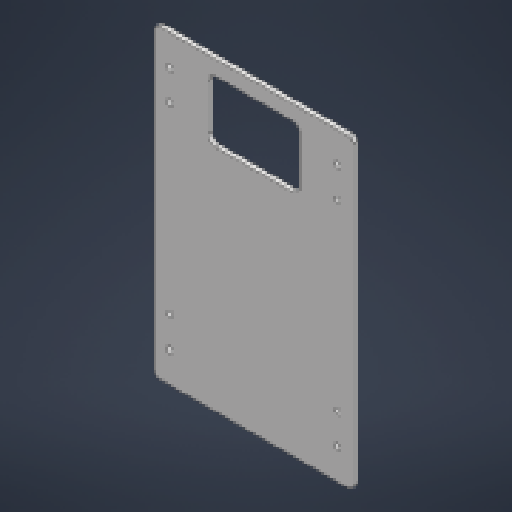
# Autodesk Inventor part: 顶板装配隔离
Saved by Autodesk Inventor 2025 (Build 290162000, 162)
## iProperties
Created: 2026-01-03
Part Number: 顶板装配隔离
Material: 常规
Document SubType Name: Modeling
Designer: XH
Density: 1 g/cm^3
Appearance: 默认
Author: XH
Autodesk Inventor part; units mm, degrees
ref_plane "YZ Plane" through (0, 0, 0) normal (1, 0, 0) x (0, 1, 0)
ref_plane "XZ Plane" through (0, 0, 0) normal (0, 1, 0) x (-1, 0, 0)
ref_plane "XY Plane" through (0, 0, 0) normal (0, 0, 1) x (1, 0, 0)
sketch "草图1" plane through (0, 0, 0) normal (0, 0, 1) x (1, 0, 0)
  line L0 (65, -50) -> (-65, -50)
  line L1 (-65, -50) -> (-65, 50)
  line L2 (-65, 50) -> (65, 50)
  line L3 (65, 50) -> (65, -50)
  line L4 (65, -50) -> (-65, 50) construction
  line L5 (-65, -50) -> (65, 50) construction
  point P0 (0, 0)
  dimension "d0" = 130
  dimension "d1" = 100
  constraints: 12 end point, 2 midpoint, 2 parallel, 1 horizontal, 1 perpendicular
  measures "d0" distance of L1.end L2.end
  measures "d1" distance of L2.end L0.start
extrude "拉伸1" add sketch "草图1" along normal blind 3
fillet "圆角1" radius 3 4 edges at (65, 50, 1.5) (65, -50, 1.5) (-65, -50, 1.5) (-65, 50, 1.5)
sketch "草图2" plane through (0, 0, 0) normal (0, 0, -1) x (-1, 0, 0)
  point P0 (0, 0)
move faces "移动1" translate (0, 50, 0) faces at (20.6667, 50, 1)
move faces "移动2" translate (0, -50, 0) faces at (-20.6667, -50, 1)
sketch "草图3" plane through (0, 0, 0) normal (0, 0, -1) x (-1, 0, 0)
  circle A0 centre (-51, -3) radius 2 projected
  circle A1 centre (51, -3) radius 2 projected
  arc A2 (35, -95) -> (40, -100) centre (40, -95) ccw projected
  line L0 (35, -95) -> (35, -55) projected
  arc A3 (35, -55) -> (30, -50) centre (30, -55) ccw projected
  line L1 (30, -50) -> (-30, -50) projected
  arc A4 (-30, -50) -> (-35, -55) centre (-30, -55) ccw projected
  line L2 (-35, -55) -> (-35, -95) projected
  arc A5 (-40, -100) -> (-35, -95) centre (-40, -95) ccw projected
  line L3 (-65, -100) -> (-40, -100) projected
  line L4 (-65, -20) -> (-65, -100) projected
  line L5 (-65, -20) -> (-120, -20) projected
  line L6 (-120, -20) -> (-120, 20) projected
  line L7 (-120, 20) -> (-65, 20) projected
  line L8 (-65, 100) -> (-65, 20) projected
  line L9 (65, 100) -> (-65, 100) projected
  line L10 (65, 20) -> (65, 100) projected
  line L11 (65, 20) -> (120, 20) projected
  line L12 (120, 20) -> (120, -20) projected
  line L13 (120, -20) -> (65, -20) projected
  line L14 (65, -100) -> (65, -20) projected
  line L15 (40, -100) -> (65, -100) projected
  line L16 (-25, 50) -> (25, 50) projected
  arc A6 (25, 50) -> (30, 55) centre (25, 55) ccw projected
  line L17 (30, 55) -> (30, 85) projected
  arc A7 (30, 85) -> (25, 90) centre (25, 85) ccw projected
  line L18 (25, 90) -> (-25, 90) projected
  arc A8 (-25, 90) -> (-30, 85) centre (-25, 85) ccw projected
  line L19 (-30, 85) -> (-30, 55) projected
  arc A9 (-30, 55) -> (-25, 50) centre (-25, 55) ccw projected
  circle A10 centre (-106, -10) radius 2.5 projected
  circle A11 centre (86, 10) radius 2.5 projected
  circle A12 centre (-86, -10) radius 2.5 projected
  circle A13 centre (-86, 10) radius 2.5 projected
  circle A14 centre (106, -10) radius 2.5 projected
  circle A15 centre (106, 10) radius 2.5 projected
  circle A16 centre (-106, 10) radius 2.5 projected
  circle A17 centre (86, -10) radius 2.5 projected
  line L20 (-8.0092, 23.9084) -> (-13.0092, 23.9084) projected
  line L21 (-13.0092, 23.9084) -> (-13.0092, 18.9084) projected
  line L22 (-13.0092, 18.9084) -> (-8.0092, 18.9084) projected
  line L23 (-8.0092, 18.9084) -> (-8.0092, 23.9084) projected
  line L24 (-23.0092, 23.9084) -> (-28.0092, 23.9084) projected
  line L25 (-28.0092, 23.9084) -> (-28.0092, 18.9084) projected
  line L26 (-28.0092, 18.9084) -> (-23.0092, 18.9084) projected
  line L27 (-23.0092, 18.9084) -> (-23.0092, 23.9084) projected
  line L28 (-8.0092, -26.0916) -> (-13.0092, -26.0916) projected
  line L29 (-13.0092, -26.0916) -> (-13.0092, -31.0916) projected
  line L30 (-13.0092, -31.0916) -> (-8.0092, -31.0916) projected
  line L31 (-8.0092, -31.0916) -> (-8.0092, -26.0916) projected
  line L32 (-23.0092, -26.0916) -> (-28.0092, -26.0916) projected
  line L33 (-28.0092, -26.0916) -> (-28.0092, -31.0916) projected
  line L34 (-28.0092, -31.0916) -> (-23.0092, -31.0916) projected
  line L35 (-23.0092, -31.0916) -> (-23.0092, -26.0916) projected
  circle A18 centre (-55, -60) radius 2 projected
  circle A19 centre (55, 60) radius 2 projected
  circle A20 centre (-55, 80) radius 2 projected
  circle A21 centre (-55, -80) radius 2 projected
  circle A22 centre (55, -80) radius 2 projected
  circle A23 centre (55, 80) radius 2 projected
  circle A24 centre (-55, 60) radius 2 projected
  circle A25 centre (55, -60) radius 2 projected
  point P0 (0, 0)
extrude "拉伸2" cut sketch "草图3" against normal blind 10 contours A9 L19 A8 L18 A7 L17 A6 L16
sketch "草图4" plane through (0, 0, 0) normal (0, 0, -1) x (-1, 0, 0)
  circle A0 centre (-55, -60) radius 2 construction
  circle A1 centre (55, 60) radius 2 construction
  circle A2 centre (-55, 80) radius 2 construction
  circle A3 centre (-55, -80) radius 2 construction
  circle A4 centre (55, -80) radius 2 construction
  circle A5 centre (55, 80) radius 2 construction
  circle A6 centre (-55, 60) radius 2 construction
  circle A7 centre (55, -60) radius 2 construction
  line L0 (-8.0092, 23.9084) -> (-13.0092, 23.9084) construction
  line L1 (-13.0092, 23.9084) -> (-13.0092, 18.9084) construction
  line L2 (-13.0092, 18.9084) -> (-8.0092, 18.9084) construction
  line L3 (-8.0092, 18.9084) -> (-8.0092, 23.9084) construction
  line L4 (-23.0092, 23.9084) -> (-28.0092, 23.9084) construction
  line L5 (-28.0092, 23.9084) -> (-28.0092, 18.9084) construction
  line L6 (-28.0092, 18.9084) -> (-23.0092, 18.9084) construction
  line L7 (-23.0092, 18.9084) -> (-23.0092, 23.9084) construction
  line L8 (-8.0092, -26.0916) -> (-13.0092, -26.0916) construction
  line L9 (-13.0092, -26.0916) -> (-13.0092, -31.0916) construction
  line L10 (-13.0092, -31.0916) -> (-8.0092, -31.0916) construction
  line L11 (-8.0092, -31.0916) -> (-8.0092, -26.0916) construction
  line L12 (-23.0092, -26.0916) -> (-28.0092, -26.0916) construction
  line L13 (-28.0092, -26.0916) -> (-28.0092, -31.0916) construction
  line L14 (-28.0092, -31.0916) -> (-23.0092, -31.0916) construction
  line L15 (-23.0092, -31.0916) -> (-23.0092, -26.0916) construction
  circle A8 centre (-51, -3) radius 2 construction
  circle A9 centre (51, -3) radius 2 construction
  arc A10 (35, -95) -> (40, -100) centre (40, -95) ccw construction
  line L16 (35, -95) -> (35, -55) construction
  arc A11 (35, -55) -> (30, -50) centre (30, -55) ccw construction
  line L17 (30, -50) -> (-30, -50) construction
  arc A12 (-30, -50) -> (-35, -55) centre (-30, -55) ccw construction
  line L18 (-35, -55) -> (-35, -95) construction
  arc A13 (-40, -100) -> (-35, -95) centre (-40, -95) ccw construction
  line L19 (-65, -100) -> (-40, -100) construction
  line L20 (-65, -20) -> (-65, -100) construction
  line L21 (-65, -20) -> (-120, -20) construction
  line L22 (-120, -20) -> (-120, 20) construction
  line L23 (-120, 20) -> (-65, 20) construction
  line L24 (-65, 100) -> (-65, 20) construction
  line L25 (65, 100) -> (-65, 100) construction
  line L26 (65, 20) -> (65, 100) construction
  line L27 (65, 20) -> (120, 20) construction
  line L28 (120, 20) -> (120, -20) construction
  line L29 (120, -20) -> (65, -20) construction
  line L30 (65, -100) -> (65, -20) construction
  line L31 (40, -100) -> (65, -100) construction
  line L32 (-25, 50) -> (25, 50) construction
  arc A14 (25, 50) -> (30, 55) centre (25, 55) ccw construction
  line L33 (30, 55) -> (30, 85) construction
  arc A15 (30, 85) -> (25, 90) centre (25, 85) ccw construction
  line L34 (25, 90) -> (-25, 90) construction
  arc A16 (-25, 90) -> (-30, 85) centre (-25, 85) ccw construction
  line L35 (-30, 85) -> (-30, 55) construction
  arc A17 (-30, 55) -> (-25, 50) centre (-25, 55) ccw construction
  circle A18 centre (-106, -10) radius 2.5 construction
  circle A19 centre (86, 10) radius 2.5 construction
  circle A20 centre (-86, -10) radius 2.5 construction
  circle A21 centre (-86, 10) radius 2.5 construction
  circle A22 centre (106, -10) radius 2.5 construction
  circle A23 centre (106, 10) radius 2.5 construction
  circle A24 centre (-106, 10) radius 2.5 construction
  circle A25 centre (86, -10) radius 2.5 construction
  circle A26 centre (-55, 80) radius 2 projected
  circle A27 centre (-55, 60) radius 2 projected
  circle A28 centre (-55, -60) radius 2 projected
  circle A29 centre (-55, -80) radius 2 projected
  circle A30 centre (55, -80) radius 2 projected
  circle A31 centre (55, -60) radius 2 projected
  circle A32 centre (55, 60) radius 2 projected
  circle A33 centre (55, 80) radius 2 projected
  point P0 (0, 0)
extrude "拉伸3" cut sketch "草图4" against normal blind 10
